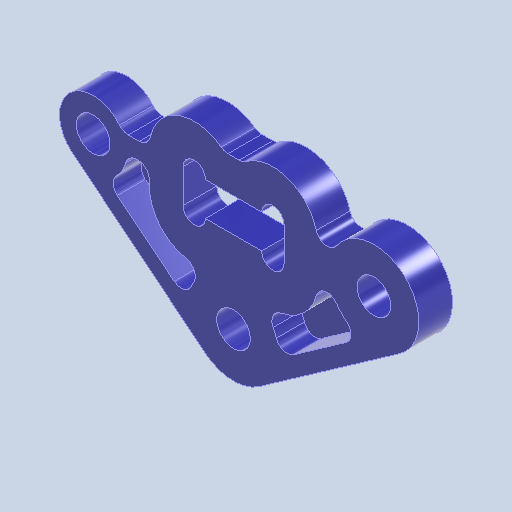
# Autodesk Inventor part: 足 横wing固定用外フレーム
Saved by Autodesk Inventor 2023.1 (Build 271208000, 208)
## iProperties
Created: 2020-05-17
Part Number: 足 横wing固定用外フレーム
Material: アルミニウム 2014-T6
Document SubType Name: Modeling
Designer: mozar
Density: 2.78927 g/cm^3
Appearance: 滑らか - 濃紺色
Mass: 2.27772 g
Surface Area: 11.4754 cm^2
Volume: 0.8166 cm^3
Author: mozar
Autodesk Inventor part; units mm, degrees
ref_plane "YZ Plane" through (0, 0, 0) normal (1, 0, 0) x (0, 1, 0)
ref_plane "XZ Plane" through (0, 0, 0) normal (0, 1, 0) x (-1, 0, 0)
ref_plane "XY Plane" through (0, 0, 0) normal (0, 0, 1) x (1, 0, 0)
sketch "スケッチ1" plane through (0, 0, 0) normal (0, 0, 1) x (1, 0, 0)
  arc A0 (-67.3471, 114.501) -> (-65.1952, 116.9091) centre (-69, 118.1435) ccw
  line L0 (-67.3471, 114.501) -> (-45.8039, 94.0088)
  line L1 (-45.8039, 94.0088) -> (-41.2946, 99.2468)
  arc A1 (-42.0113, 103.4843) -> (-41.2946, 99.2468) centre (-38.3264, 101.9283) ccw
  line L2 (-42.0113, 103.4843) -> (-65.1952, 116.9091)
  circle A2 centre (-69, 118.1435) radius 1.5
  line L3 (-8.5314, 132.4283) -> (8.5314, 132.4283)
  arc A3 (8.9906, 133.8477) -> (8.5314, 132.4283) centre (12.5, 131.9283) ccw
  line L4 (8.9906, 133.8477) -> (-8.0073, 147.851)
  arc A4 (-12.2806, 145.8755) -> (-8.0073, 147.851) centre (-12.9215, 152.8712) ccw
  line L5 (-12.2806, 145.8755) -> (-12.08, 135.9062)
  arc A5 (-8.5314, 132.4283) -> (-12.08, 135.9062) centre (-12.5, 131.9283) ccw
  line L6 (-40.5367, 98.5944) -> (-45.0784, 93.3188)
  line L7 (-45.0784, 93.3188) -> (-23.1821, 72.4907)
  arc A6 (-21.219, 73.2225) -> (-23.1821, 72.4907) centre (-20.8522, 69.2393) ccw
  line L8 (-21.219, 73.2225) -> (-20.9998, 79.7658)
  arc A7 (-26.8226, 92.2649) -> (-20.9998, 79.7658) centre (-20.2328, 87.729) ccw
  line L9 (-26.8226, 92.2649) -> (-35.513, 99.0849)
  arc A8 (-40.5367, 98.5944) -> (-35.513, 99.0849) centre (-38.3264, 101.9283) ccw
  line L10 (-53.762, 124.0122) -> (-40.2555, 105.4324)
  arc A9 (-36.7463, 105.603) -> (-40.2555, 105.4324) centre (-38.3264, 101.9283) ccw
  arc A10 (-36.7463, 105.603) -> (-35.5935, 105.8692) centre (-36.3513, 106.5217) ccw
  line L11 (-35.5935, 105.8692) -> (-15.9908, 128.6398)
  arc A11 (-15.9908, 128.6398) -> (-15.8989, 129.8194) centre (-16.7486, 129.2922) ccw
  arc A12 (-16.3868, 130.9834) -> (-15.8989, 129.8194) centre (-12.5, 131.9283) ccw
  line L12 (-16.3868, 130.9834) -> (-52.5003, 126.8796)
  arc A13 (-53.762, 124.0122) -> (-52.5003, 126.8796) centre (-56.5, 126.9283) ccw
  line L13 (-20.101, 159.5757) -> (-51.6361, 130.4057)
  line L14 (-51.6361, 130.4057) -> (-19.1983, 149.7164)
  arc A14 (-18.3334, 157.3502) -> (-19.1983, 149.7164) centre (-12.9215, 152.8712) ccw
  arc A15 (-18.3334, 157.3502) -> (-18.8282, 158.9491) centre (-19.1038, 157.9878) ccw
  arc A16 (-20.101, 159.5757) -> (-18.8282, 158.9491) centre (-17.726, 162.7942) ccw
  line L15 (-52.6132, 127.8732) -> (-16.4997, 131.977)
  arc A17 (-13.0798, 135.886) -> (-16.4997, 131.977) centre (-12.5, 131.9283) ccw
  line L16 (-13.0798, 135.886) -> (-13.2804, 145.8553)
  arc A18 (-18.6867, 148.8571) -> (-13.2804, 145.8553) centre (-12.9215, 152.8712) ccw
  line L17 (-18.6867, 148.8571) -> (-52.8341, 128.5287)
  arc A19 (-52.6132, 127.8732) -> (-52.8341, 128.5287) centre (-56.5, 126.9283) ccw
  line L18 (-41.0644, 104.8444) -> (-54.5709, 123.4242)
  arc A20 (-57.3125, 123.0117) -> (-54.5709, 123.4242) centre (-56.5, 126.9283) ccw
  arc A21 (-63.1458, 122.4283) -> (-57.3125, 123.0117) centre (-60.5, 125.4283) ccw
  line L19 (-63.1458, 122.4283) -> (-66.7175, 122.4283)
  arc A22 (-66.7175, 122.4283) -> (-67.6036, 121.8918) centre (-66.7175, 121.4283) ccw
  arc A23 (-65.0045, 117.9542) -> (-67.6036, 121.8918) centre (-69, 118.1435) ccw
  line L20 (-65.0045, 117.9542) -> (-41.5102, 104.3497)
  arc A24 (-41.0644, 104.8444) -> (-41.5102, 104.3497) centre (-38.3264, 101.9283) ccw
  circle A25 centre (20.2328, 87.729) radius 5.75
  circle A26 centre (-20.2328, 87.729) radius 5.75
  circle A27 centre (-20.8522, 69.2393) radius 1.5
  circle A28 centre (-19.5, 53.0338) radius 1.5
  line L21 (-19.7781, 65.3862) -> (-19.5876, 63.104)
  line L22 (-19.5876, 63.104) -> (-7.2173, 67.5101)
  arc A29 (-5.9007, 74.1795) -> (-7.2173, 67.5101) centre (0, 69.55) ccw
  line L23 (-5.9007, 74.1795) -> (-14.6278, 82.0207)
  arc A30 (-20.0004, 79.7323) -> (-14.6278, 82.0207) centre (-20.2328, 87.729) ccw
  line L24 (-20.0004, 79.7323) -> (-20.2196, 73.189)
  arc A31 (-19.7781, 65.3862) -> (-20.2196, 73.189) centre (-20.8522, 69.2393) ccw
  circle A32 centre (-17.726, 162.7942) radius 1.5
  circle A33 centre (-12.9215, 152.8712) radius 4.025
  line L25 (-34.7337, 103.6868) -> (-0.8086, 115.3011)
  line L26 (-0.8086, 115.3011) -> (-10.5399, 128.4414)
  arc A34 (-14.0801, 128.2536) -> (-10.5399, 128.4414) centre (-12.5, 131.9283) ccw
  arc A35 (-14.0801, 128.2536) -> (-15.2329, 127.9873) centre (-14.4751, 127.3349) ccw
  line L27 (-15.2329, 127.9873) -> (-34.8356, 105.2168)
  arc A36 (-34.8356, 105.2168) -> (-34.9275, 104.0372) centre (-34.0778, 104.5644) ccw
  arc A37 (-34.7337, 103.6868) -> (-34.9275, 104.0372) centre (-38.3264, 101.9283) ccw
  line L28 (0.8086, 115.3011) -> (34.7337, 103.6868)
  arc A38 (35.1946, 104.4166) -> (34.7337, 103.6868) centre (38.3264, 101.9283) ccw
  line L29 (35.1946, 104.4166) -> (14.9874, 127.8894)
  arc A39 (14.9874, 127.8894) -> (13.8836, 128.1752) centre (14.2295, 127.2369) ccw
  arc A40 (10.5399, 128.4414) -> (13.8836, 128.1752) centre (12.5, 131.9283) ccw
  line L30 (10.5399, 128.4414) -> (0.8086, 115.3011)
  line L31 (34.4098, 102.7407) -> (1.3578, 114.0561)
  line L32 (1.3578, 114.0561) -> (15.8828, 94.4429)
  arc A41 (26.2052, 93.0515) -> (15.8828, 94.4429) centre (20.2328, 87.729) ccw
  line L33 (26.2052, 93.0515) -> (34.8957, 99.8715)
  arc A42 (34.4098, 102.7407) -> (34.8957, 99.8715) centre (38.3264, 101.9283) ccw
  line L34 (0, 114.2093) -> (-15.0792, 93.8478)
  arc A43 (-12.2484, 88.229) -> (-15.0792, 93.8478) centre (-20.2328, 87.729) ccw
  line L35 (-12.2484, 88.229) -> (12.2484, 88.229)
  arc A44 (15.0792, 93.8478) -> (12.2484, 88.229) centre (20.2328, 87.729) ccw
  line L36 (15.0792, 93.8478) -> (0, 114.2093)
  line L37 (0, 115.8896) -> (9.7363, 129.0366)
  arc A45 (8.753, 130.5283) -> (9.7363, 129.0366) centre (12.5, 131.9283) ccw
  arc A46 (8.753, 130.5283) -> (7.8163, 131.1783) centre (7.8163, 130.1783) ccw
  line L38 (7.8163, 131.1783) -> (-7.8163, 131.1783)
  arc A47 (-7.8163, 131.1783) -> (-8.753, 130.5283) centre (-7.8163, 130.1783) ccw
  arc A48 (-9.7363, 129.0366) -> (-8.753, 130.5283) centre (-12.5, 131.9283) ccw
  line L39 (-9.7363, 129.0366) -> (0, 115.8896)
  circle A49 centre (-12.5, 131.9283) radius 1.5
  line L40 (-34.8957, 99.8715) -> (-26.2052, 93.0515)
  arc A50 (-15.8828, 94.4429) -> (-26.2052, 93.0515) centre (-20.2328, 87.729) ccw
  line L41 (-15.8828, 94.4429) -> (-1.3578, 114.0561)
  line L42 (-1.3578, 114.0561) -> (-34.4098, 102.7407)
  arc A51 (-34.8957, 99.8715) -> (-34.4098, 102.7407) centre (-38.3264, 101.9283) ccw
  line L43 (42.9737, 57.5032) -> (38.0562, 97.9374)
  arc A52 (35.513, 99.0849) -> (38.0562, 97.9374) centre (38.3264, 101.9283) ccw
  line L44 (35.513, 99.0849) -> (26.8226, 92.2649)
  arc A53 (25.202, 81.4595) -> (26.8226, 92.2649) centre (20.2328, 87.729) ccw
  line L45 (25.202, 81.4595) -> (42.111, 57.1462)
  arc A54 (42.9737, 57.5032) -> (42.111, 57.1462) centre (44.2539, 53.1892) ccw
  arc A55 (-13.9594, 82.7646) -> (-12.2484, 87.229) centre (-20.2328, 87.729) ccw
  line L46 (-13.9594, 82.7646) -> (-5.2323, 74.9234)
  arc A56 (5.2323, 74.9234) -> (-5.2323, 74.9234) centre (0, 69.55) ccw
  line L47 (5.2323, 74.9234) -> (13.9594, 82.7646)
  arc A57 (12.2484, 87.229) -> (13.9594, 82.7646) centre (20.2328, 87.729) ccw
  line L48 (12.2484, 87.229) -> (-12.2484, 87.229)
  line L49 (7.1924, 67.424) -> (40.2326, 55.2089)
  arc A58 (41.29, 56.5752) -> (40.2326, 55.2089) centre (44.2539, 53.1892) ccw
  line L50 (41.29, 56.5752) -> (24.381, 80.8885)
  arc A59 (14.6278, 82.0207) -> (24.381, 80.8885) centre (20.2328, 87.729) ccw
  line L51 (14.6278, 82.0207) -> (5.9007, 74.1795)
  arc A60 (7.1924, 67.424) -> (5.9007, 74.1795) centre (0, 69.55) ccw
  circle A61 centre (0, 69.55) radius 4.5
  arc A62 (-1.9, 54.6661) -> (-0.5, 55.5826) centre (-1.5, 55.5826) ccw
  line L52 (-0.5, 55.5826) -> (-0.5, 61.1834)
  arc A63 (-0.5, 61.1834) -> (-1.3235, 62.1677) centre (-1.5, 61.1834) ccw
  arc A64 (-6.8817, 66.5681) -> (-1.3235, 62.1677) centre (0, 69.55) ccw
  line L53 (-6.8817, 66.5681) -> (-19.5016, 62.0731)
  line L54 (-19.5016, 62.0731) -> (-19.0793, 57.0116)
  arc A65 (-15.8112, 51.487) -> (-19.0793, 57.0116) centre (-19.5, 53.0338) ccw
  arc A66 (-15.8112, 51.487) -> (-11.0422, 51.0882) centre (-7.5, 122.1642) ccw
  arc A67 (-8.1719, 51.9865) -> (-11.0422, 51.0882) centre (-8.5, 48) ccw
  arc A68 (-8.1719, 51.9865) -> (-7.1719, 52.5865) centre (-8.0899, 52.9832) ccw
  arc A69 (-1.9, 54.6661) -> (-7.1719, 52.5865) centre (-3.5, 51) ccw
  circle A70 centre (44.2539, 53.1892) radius 1.5
  arc A71 (10.9, 51.2) -> (11.5, 51) centre (11.5, 52) ccw
  line L55 (11.5, 51) -> (11.6438, 51)
  arc A72 (11.6438, 51) -> (12.2438, 51.2) centre (11.6438, 52) ccw
  arc A73 (14.9719, 51.9865) -> (12.2438, 51.2) centre (14.6438, 48) ccw
  arc A74 (14.9719, 51.9865) -> (15.9719, 52.5865) centre (15.0539, 52.9832) ccw
  arc A75 (22.2896, 54) -> (15.9719, 52.5865) centre (19.6438, 51) ccw
  line L56 (22.2896, 54) -> (23.9981, 54)
  arc A76 (30.5528, 51.8483) -> (23.9981, 54) centre (26.6438, 51) ccw
  arc A77 (33.5683, 51.5066) -> (30.5528, 51.8483) centre (31.6438, 48) ccw
  arc A78 (33.5683, 51.5066) -> (34.4381, 51) centre (34.4381, 52) ccw
  line L57 (34.4381, 51) -> (35.1308, 51)
  arc A79 (35.1308, 51) -> (35.5246, 51.0808) centre (35.1308, 52) ccw
  line L58 (35.5246, 51.0808) -> (39.1601, 52.6385)
  arc A80 (39.1601, 52.6385) -> (39.764, 53.4907) centre (38.7663, 53.5577) ccw
  arc A81 (39.8859, 54.271) -> (39.764, 53.4907) centre (44.2539, 53.1892) ccw
  line L59 (39.8859, 54.271) -> (6.8456, 66.4861)
  arc A82 (1.3235, 62.1677) -> (6.8456, 66.4861) centre (0, 69.55) ccw
  arc A83 (1.3235, 62.1677) -> (0.5, 61.1834) centre (1.5, 61.1834) ccw
  line L60 (0.5, 61.1834) -> (0.5, 55.5826)
  arc A84 (0.5, 55.5826) -> (1.9, 54.6661) centre (1.5, 55.5826) ccw
  arc A85 (7.1719, 52.5865) -> (1.9, 54.6661) centre (3.5, 51) ccw
  arc A86 (7.1719, 52.5865) -> (8.1719, 51.9865) centre (8.0899, 52.9832) ccw
  arc A87 (10.9, 51.2) -> (8.1719, 51.9865) centre (8.5, 48) ccw
  arc A88 (9.5, 48) -> (7.5, 48) centre (8.5, 48) ccw
  line L61 (7.5, 48) -> (7.5, 45)
  line L62 (7.5, 45) -> (-7.5, 45)
  line L63 (-7.5, 45) -> (-7.5, 48)
  arc A89 (-7.5, 48) -> (-9.4996, 48.027) centre (-8.5, 48) ccw
  arc A90 (-20.1841, 49.0927) -> (-9.4996, 48.027) centre (-7.5, 122.1642) ccw
  arc A91 (-20.5741, 56.8869) -> (-20.1841, 49.0927) centre (-19.5, 53.0338) ccw
  line L64 (-20.5741, 56.8869) -> (-21.2729, 65.2615)
  arc A92 (-24.2159, 71.4039) -> (-21.2729, 65.2615) centre (-20.8522, 69.2393) ccw
  line L65 (-24.2159, 71.4039) -> (-69.1506, 114.1463)
  arc A93 (-72.9846, 117.7933) -> (-69.1506, 114.1463) centre (-69, 118.1435) ccw
  line L66 (-72.9846, 117.7933) -> (-76.8602, 121.4798)
  arc A94 (-81.2136, 123.942) -> (-76.8602, 121.4798) centre (-77.5, 125.4283) ccw
  arc A95 (-81.2136, 129.9146) -> (-81.2136, 123.942) centre (-81.5, 126.9283) ccw
  arc A96 (-74.8542, 131.4283) -> (-81.2136, 129.9146) centre (-77.5, 128.4283) ccw
  line L67 (-74.8542, 131.4283) -> (-63.1458, 131.4283)
  arc A97 (-57.3125, 130.8449) -> (-63.1458, 131.4283) centre (-60.5, 128.4283) ccw
  arc A98 (-54.125, 130.1469) -> (-57.3125, 130.8449) centre (-56.5, 126.9283) ccw
  line L68 (-54.125, 130.1469) -> (-21.1196, 160.6768)
  arc A99 (-14.0261, 161.2742) -> (-21.1196, 160.6768) centre (-17.726, 162.7942) ccw
  arc A100 (-14.0261, 161.2742) -> (-13.0787, 159.8944) centre (-13.1011, 160.8942) ccw
  arc A101 (-7.0536, 149.0088) -> (-13.0787, 159.8944) centre (-12.9215, 152.8712) ccw
  line L69 (-7.0536, 149.0088) -> (9.9444, 135.0054)
  arc A102 (16.0056, 130.002) -> (9.9444, 135.0054) centre (12.5, 131.9283) ccw
  arc A103 (16.0056, 130.002) -> (16.1242, 128.868) centre (16.882, 129.5204) ccw
  line L70 (16.1242, 128.868) -> (35.839, 105.9672)
  arc A104 (35.839, 105.9672) -> (36.9428, 105.6814) centre (36.5969, 106.6196) ccw
  arc A105 (39.5453, 98.1185) -> (36.9428, 105.6814) centre (38.3264, 101.9283) ccw
  line L71 (39.5453, 98.1185) -> (44.4627, 57.6843)
  arc A106 (41.3752, 49.7304) -> (44.4627, 57.6843) centre (44.2539, 53.1892) ccw
  arc A107 (41.3752, 49.7304) -> (40.3416, 49.881) centre (40.7355, 48.9618) ccw
  line L72 (40.3416, 49.881) -> (36.2346, 48.1212)
  arc A108 (35.6438, 48) -> (36.2346, 48.1212) centre (35.6438, 49.5) ccw
  line L73 (35.6438, 48) -> (32.6438, 48)
  arc A109 (32.6438, 48) -> (30.6438, 48) centre (31.6438, 48) ccw
  line L74 (30.6438, 48) -> (30.6438, 45)
  line L75 (30.6438, 45) -> (15.6438, 45)
  line L76 (15.6438, 45) -> (15.6438, 48)
  arc A110 (15.6438, 48) -> (13.6438, 48) centre (14.6438, 48) ccw
  line L77 (13.6438, 48) -> (9.5, 48)
  line L78 (18.6438, 51) -> (18.6438, 48)
  arc A111 (18.6438, 48) -> (20.6438, 48) centre (19.6438, 48) ccw
  line L79 (20.6438, 48) -> (25.6438, 48)
  arc A112 (25.6438, 48) -> (27.6438, 48) centre (26.6438, 48) ccw
  line L80 (27.6438, 48) -> (27.6438, 51)
  arc A113 (27.6438, 51) -> (25.6438, 51) centre (26.6438, 51) ccw
  line L81 (25.6438, 51) -> (20.6438, 51)
  arc A114 (20.6438, 51) -> (18.6438, 51) centre (19.6438, 51) ccw
  line L82 (-4.5, 51) -> (-4.5, 48)
  arc A115 (-4.5, 48) -> (-2.5, 48) centre (-3.5, 48) ccw
  line L83 (-2.5, 48) -> (2.5, 48)
  arc A116 (2.5, 48) -> (4.5, 48) centre (3.5, 48) ccw
  line L84 (4.5, 48) -> (4.5, 51)
  arc A117 (4.5, 51) -> (2.5, 51) centre (3.5, 51) ccw
  line L85 (2.5, 51) -> (-2.5, 51)
  arc A118 (-2.5, 51) -> (-4.5, 51) centre (-3.5, 51) ccw
  circle A119 centre (12.5, 131.9283) radius 1.5
  circle A120 centre (-38.3264, 101.9283) radius 1.5
  circle A121 centre (38.3264, 101.9283) radius 1.5
  arc A122 (42.1775, 57.1816) -> (42.1571, 57.1709) centre (44.2546, 53.1897) ccw
  line L86 (42.1571, 57.1709) -> (42.1563, 57.1713)
  arc A123 (42.1563, 57.1713) -> (42.1775, 57.1816) centre (41.7307, 58.0762) ccw
  circle A124 centre (-56.5, 126.9283) radius 1.5
  circle A125 centre (-81.5, 126.9283) radius 1.5
  line L87 (-78.5, 128.4283) -> (-78.5, 125.4283)
  arc A126 (-78.5, 125.4283) -> (-76.5, 125.4283) centre (-77.5, 125.4283) ccw
  line L88 (-76.5, 125.4283) -> (-61.5, 125.4283)
  arc A127 (-61.5, 125.4283) -> (-59.5, 125.4283) centre (-60.5, 125.4283) ccw
  line L89 (-59.5, 125.4283) -> (-59.5, 128.4283)
  arc A128 (-59.5, 128.4283) -> (-61.5, 128.4283) centre (-60.5, 128.4283) ccw
  line L90 (-61.5, 128.4283) -> (-76.5, 128.4283)
  arc A129 (-76.5, 128.4283) -> (-78.5, 128.4283) centre (-77.5, 128.4283) ccw
  line L91 (-69, 118.1435) -> (-56.5, 126.9283) construction
  line L92 (-68.5688, 117.5298) -> (-56.0688, 126.3147)
  line L93 (-56.9312, 127.5419) -> (-69.4312, 118.7571)
  arc A130 (-69.4312, 118.7571) -> (-68.5688, 117.5298) centre (-69, 118.1435) ccw
  arc A131 (-56.0688, 126.3147) -> (-56.9312, 127.5419) centre (-56.5, 126.9283) ccw
  line L94 (-81.5, 126.9283) -> (-69, 118.1435) construction
  line L95 (-81.9312, 126.3147) -> (-69.4312, 117.5298)
  line L96 (-68.5688, 118.7571) -> (-81.0688, 127.5419)
  arc A132 (-81.0688, 127.5419) -> (-81.9312, 126.3147) centre (-81.5, 126.9283) ccw
  arc A133 (-69.4312, 117.5298) -> (-68.5688, 118.7571) centre (-69, 118.1435) ccw
  line L97 (-63.1458, 122.4283) -> (-74.8542, 122.4283)
  arc A134 (-81.5, 125.4283) -> (-74.8542, 122.4283) centre (-77.5, 125.4283) ccw
  line L98 (-81.5, 125.4283) -> (-81.5, 128.4283)
  arc A135 (-74.8542, 131.4283) -> (-81.5, 128.4283) centre (-77.5, 128.4283) ccw
  line L99 (-74.8542, 131.4283) -> (-63.1458, 131.4283)
  arc A136 (-56.5, 128.4283) -> (-63.1458, 131.4283) centre (-60.5, 128.4283) ccw
  line L100 (-56.5, 128.4283) -> (-56.5, 125.4283)
  arc A137 (-63.1458, 122.4283) -> (-56.5, 125.4283) centre (-60.5, 125.4283) ccw
  circle A138 centre (-56.5, 126.9283) radius 4
  circle A139 centre (-69, 118.1435) radius 4
  point P0 (0, 0)
  point P1 (0, 0)
  point P2 (-62.75, 122.5359)
  point P3 (-75.25, 122.5359)
  point P4 (-62.3651, 121.8897)
  point P5 (-75.6349, 121.8897)
  point P6 (-72.6458, 119.789)
  point P7 (-67.3471, 114.501)
  point P8 (-65.1952, 116.9091)
  point P9 (-65.3542, 119.789)
  dimension "d0" = 1.5
  dimension "d1" = 1.5
  dimension "d2" = 3
  constraints: 246 point on circle, 206 end point, 138 centre point, 19 horizontal, 12 vertical, 8 tangent, 2 coincident, 2 midpoint, 2 parallel, 1 concentric, 541 other
  measures "d0" diameter of A131
  measures "d1" diameter of A133
  measures "d2" distance between parallel lines of L88 L97
extrude "押し出し2" add sketch "スケッチ1" against normal blind 3 contours A139 A93 L95 A2 L92 A23 A0 | A94 A134 A125 L95 | A139 L96 A2 L95 | L95 A134 L97 L96 A139 | L92 A2 L93 A23 | A23 L93 L19 A21 L92 | A95 A135 A125 A134 | L95 A125 L96 L87 A126 L97 A134 | L95 A130 L92 A2 | A2 L96 L93 A130 L95 | A139 A23 L93 A2 L96 | L96 L97 A22 A139 | A23 A22 L19 L93 | L92 A133 L96 L93 A2 | L92 A138 A21 | A21 L19 L93 A127 A138 L92 | A20 A137 A124 A136 A98 A138 A19 A13 | A96 L67 A97 A138 A128 L90 A129 L87 L96 A125 A135 | L98 L95 A125 | A125 L98 A132 L95 | L95 L98 A132 L96 A125 | A2 L93 L96 | A130 L93 L96 A133 | L96 A126 L88 A127 L93 L19 L97 | A138 L92 A124 A137 | A138 A127 L89 L93 A124 L92 | A125 L96 A132 L98 | L95 A132 L98 | L100 L92 A131 A124 | A124 L92 L100 | A124 L93 A131 L100 L92 | L100 A131 L92 | L93 L89 A128 A138 A136 A124 | A124 L100 A131 L93
sketch "スケッチ2" plane through (0, 0, 0) normal (0, 0, 1) x (1, 0, 0)
  line L0 (-76.5, 125.4283) -> (-61.5, 125.4283) projected
  arc A0 (-61.5, 125.4283) -> (-59.5, 125.4283) centre (-60.5, 125.4283) ccw projected
  line L1 (-59.5, 125.4283) -> (-59.5, 128.4283) projected
  arc A1 (-59.5, 128.4283) -> (-61.5, 128.4283) centre (-60.5, 128.4283) ccw projected
  line L2 (-61.5, 128.4283) -> (-76.5, 128.4283) projected
  arc A2 (-76.5, 128.4283) -> (-78.5, 128.4283) centre (-77.5, 128.4283) ccw projected
  line L3 (-78.5, 128.4283) -> (-78.5, 125.4283) projected
  arc A3 (-78.5, 125.4283) -> (-76.5, 125.4283) centre (-77.5, 125.4283) ccw projected
  line L4 (-72.6458, 119.789) -> (-75.6349, 121.8897) projected
  arc A4 (-81.2136, 123.942) -> (-75.6349, 121.8897) centre (-77.5, 125.4283) ccw projected
  arc A5 (-81.2136, 129.9146) -> (-81.2136, 123.942) centre (-81.5, 126.9283) ccw projected
  arc A6 (-74.8542, 131.4283) -> (-81.2136, 129.9146) centre (-77.5, 128.4283) ccw projected
  line L5 (-74.8542, 131.4283) -> (-63.1458, 131.4283) projected
  arc A7 (-57.3125, 130.8449) -> (-63.1458, 131.4283) centre (-60.5, 128.4283) ccw projected
  arc A8 (-57.3125, 123.0117) -> (-57.3125, 130.8449) centre (-56.5, 126.9283) ccw projected
  arc A9 (-62.3651, 121.8897) -> (-57.3125, 123.0117) centre (-60.5, 125.4283) ccw projected
  line L6 (-62.3651, 121.8897) -> (-65.3542, 119.789) projected
  arc A10 (-72.6458, 119.789) -> (-65.3542, 119.789) centre (-69, 118.1435) ccw projected
  point P0 (0, 0)
hole "穴1" at (-56.5, 126.9283, 0) at (-81.5, 126.9283, 0) at (-69, 118.1435, 0) direction (0, 0, -1) diameter 3 depth 12 tip angle 118
fillet "フィレット1" radius 1 10 edges at (-62.3651, 121.8897, -1.5) (-57.3125, 123.0117, -1.5) (-65.3542, 119.789, -1.5) (-57.3125, 130.8449, -1.5) (-72.6458, 119.789, -1.5) (-75.6349, 121.8897, -1.5) (-63.1458, 131.4283, -1.5) (-81.2136, 123.942, -1.5) (-74.8542, 131.4283, -1.5) (-81.2136, 129.9146, -1.5)
sketch "スケッチ3" plane through (0, 0, 0) normal (0, 0, 1) x (1, 0, 0)
  arc A0 (-80.9707, 123.4398) -> (-81.7538, 123.939) centre (-81.8384, 122.9426) ccw projected
  arc A1 (-81.7538, 129.9175) -> (-81.7538, 123.939) centre (-81.5, 126.9283) ccw projected
  arc A2 (-81.7538, 129.9175) -> (-80.9707, 130.4168) centre (-81.8384, 130.9139) ccw projected
  arc A3 (-75.1, 131.6283) -> (-80.9707, 130.4168) centre (-77.5, 128.4283) ccw projected
  arc A4 (-75.1, 131.6283) -> (-74.5, 131.4283) centre (-74.5, 132.4283) ccw projected
  line L0 (-74.5, 131.4283) -> (-63.5, 131.4283) projected
  arc A5 (-63.5, 131.4283) -> (-62.9, 131.6283) centre (-63.5, 132.4283) ccw projected
  arc A6 (-57.6301, 131.2146) -> (-62.9, 131.6283) centre (-60.5, 128.4283) ccw projected
  arc A7 (-57.6301, 131.2146) -> (-56.8301, 130.9146) centre (-56.9126, 131.9112) ccw projected
  arc A8 (-56.8301, 122.9419) -> (-56.8301, 130.9146) centre (-56.5, 126.9283) ccw projected
  arc A9 (-56.8301, 122.9419) -> (-57.6301, 122.6419) centre (-56.9126, 121.9453) ccw projected
  arc A10 (-61.9028, 121.6823) -> (-57.6301, 122.6419) centre (-60.5, 125.4283) ccw projected
  arc A11 (-61.9028, 121.6823) -> (-62.8285, 121.564) centre (-62.2535, 120.7458) ccw projected
  line L1 (-62.8285, 121.564) -> (-64.7367, 120.223) projected
  arc A12 (-64.7367, 120.223) -> (-65.1294, 119.1525) centre (-64.1617, 119.4048) ccw projected
  arc A13 (-72.8706, 119.1525) -> (-65.1294, 119.1525) centre (-69, 118.1435) ccw projected
  arc A14 (-72.8706, 119.1525) -> (-73.2633, 120.223) centre (-73.8383, 119.4048) ccw projected
  line L2 (-73.2633, 120.223) -> (-75.1715, 121.564) projected
  arc A15 (-75.1715, 121.564) -> (-76.0972, 121.6823) centre (-75.7465, 120.7458) ccw projected
  arc A16 (-80.9707, 123.4398) -> (-76.0972, 121.6823) centre (-77.5, 125.4283) ccw projected
  circle A17 centre (-81.5, 126.9283) radius 1.5 projected
  circle A18 centre (-56.5, 126.9283) radius 1.5 projected
  circle A19 centre (-69, 118.1435) radius 1.5 projected
  line L3 (-76.5, 125.4283) -> (-61.5, 125.4283) projected
  arc A20 (-61.5, 125.4283) -> (-59.5, 125.4283) centre (-60.5, 125.4283) ccw projected
  line L4 (-59.5, 125.4283) -> (-59.5, 128.4283) projected
  arc A21 (-59.5, 128.4283) -> (-61.5, 128.4283) centre (-60.5, 128.4283) ccw projected
  line L5 (-61.5, 128.4283) -> (-76.5, 128.4283) projected
  arc A22 (-76.5, 128.4283) -> (-78.5, 128.4283) centre (-77.5, 128.4283) ccw projected
  line L6 (-78.5, 128.4283) -> (-78.5, 125.4283) projected
  arc A23 (-78.5, 125.4283) -> (-76.5, 125.4283) centre (-77.5, 125.4283) ccw projected
  line L7 (-76.5, 128.4283) -> (-61.5, 128.4283) projected
  line L8 (-73.5, 128.4283) -> (-64.5, 128.4283)
  line L9 (-64.5, 128.4283) -> (-64.5, 125.4283)
  line L10 (-64.5, 125.4283) -> (-73.5, 125.4283)
  line L11 (-73.5, 125.4283) -> (-73.5, 128.4283)
  circle A24 centre (-72.5, 128.4283) radius 1
  circle A25 centre (-65.5, 128.4283) radius 1
  circle A26 centre (-65.5, 125.4283) radius 1
  line L12 (-61.5, 125.4283) -> (-76.5, 125.4283) projected
  circle A27 centre (-72.5, 125.4283) radius 1
  line L13 (-61.5, 131.4283) -> (-76.5, 131.4283)
  line L14 (-76.5, 131.4283) -> (-76.5, 122.4283)
  line L15 (-76.5, 122.4283) -> (-61.5, 122.4283)
  line L16 (-61.5, 122.4283) -> (-61.5, 131.4283)
  circle A28 centre (-72.5, 128.4283) radius 4
  circle A29 centre (-65.5, 128.4283) radius 4
  circle A30 centre (-72.5, 125.4283) radius 4
  circle A31 centre (-65.5, 125.4283) radius 4
  arc A32 (-81.7538, 129.9175) -> (-81.7538, 123.939) centre (-81.5, 126.9283) ccw projected
  circle A33 centre (-81.5, 126.9283) radius 3
  circle A34 centre (-69, 118.1435) radius 4
  line L17 (-81.5, 126.9283) -> (-69, 118.1435) construction
  line L18 (-81.9312, 126.3147) -> (-69.4312, 117.5298)
  line L19 (-68.5688, 118.7571) -> (-81.0688, 127.5419)
  arc A35 (-81.0688, 127.5419) -> (-81.9312, 126.3147) centre (-81.5, 126.9283) ccw
  arc A36 (-69.4312, 117.5298) -> (-68.5688, 118.7571) centre (-69, 118.1435) ccw
  line L20 (-69, 118.1435) -> (-56.5, 126.9283) construction
  line L21 (-68.5688, 117.5298) -> (-56.0688, 126.3147)
  line L22 (-56.9312, 127.5419) -> (-69.4312, 118.7571)
  arc A37 (-69.4312, 118.7571) -> (-68.5688, 117.5298) centre (-69, 118.1435) ccw
  arc A38 (-56.0688, 126.3147) -> (-56.9312, 127.5419) centre (-56.5, 126.9283) ccw
  circle A39 centre (-81.5, 126.9283) radius 1.5 projected
  line L23 (-56.5, 126.9283) -> (-81.5, 126.9283) construction
  line L24 (-56.5, 128.4283) -> (-81.5, 128.4283)
  line L25 (-81.5, 125.4283) -> (-56.5, 125.4283)
  arc A40 (-56.5, 125.4283) -> (-56.5, 128.4283) centre (-56.5, 126.9283) ccw
  arc A41 (-81.5, 128.4283) -> (-81.5, 125.4283) centre (-81.5, 126.9283) ccw
  arc A42 (-56.8301, 122.9419) -> (-56.8301, 130.9146) centre (-56.5, 126.9283) ccw projected
  circle A43 centre (-56.5, 126.9283) radius 4
  point P0 (0, 0)
  point P1 (-69, 128.4283)
  point P2 (-75.25, 122.5359)
  point P3 (-62.75, 122.5359)
  point P4 (-69, 126.9283)
  point P5 (-63.0084, 131.5575)
  point P6 (-59.8191, 129.1607)
  point P7 (-78.9019, 128.4283)
  point P8 (-74.9916, 131.5575)
  point P9 (-79.5547, 124.6445)
  point P10 (-59.2834, 124.0555)
  point P11 (-61.5, 122.4977)
  point P12 (-61.5987, 122.4283)
  point P13 (-62.8285, 121.564)
  point P14 (-68.1458, 131.4283)
  point P15 (-69.8542, 131.4283)
  point P16 (-60.2081, 128.4283)
  dimension "d15" = 9
  dimension "d16" = 3
  dimension "d17" = 2
  dimension "d18" = 2
  dimension "d19" = 2
  dimension "d20" = 2
  dimension "d21" = 3
  dimension "d22" = 3
  dimension "d23" = 3
  dimension "d24" = 3
  dimension "d25" = 3
  dimension "d26" = 1.5
  dimension "d27" = 1.5
  dimension "d28" = 3
  constraints: 40 end point, 16 tangent, 14 centre point, 12 point on circle, 7 parallel, 5 midpoint, 5 point on line, 3 coincident, 2 horizontal, 2 perpendicular, 12 other
  measures "d15" distance of L9.end L10.end
  measures "d16" distance of L8.end L9.end
  measures "d17" diameter of A24
  measures "d18" diameter of A25
  measures "d19" diameter of A26
  measures "d20" diameter of A27
  measures "d21" distance between parallel lines of L8 L13
  measures "d22" radial gap between concentric circles of A24 A28
  measures "d23" radial gap between concentric circles of A25 A29
  measures "d24" radial gap between concentric circles of A27 A30
  measures "d25" radial gap between concentric circles of A26 A31
  measures "d26" diameter of A36
  measures "d27" diameter of A38
  measures "d28" diameter of A41
extrude "押し出し3" cut sketch "スケッチ3" against normal blind 10 contours A0 A33 L18 L14 L15 A15 A16 | A2 A3 A4 A28 L13 L14 A22 L24 A33 | L18 L15 L14 | L14 L13 A28 | A5 A6 A7 A43 A21 L16 L13 A29 | L21 L15 L16 A43 A9 A10 A11 | L13 L16 A29
extrude "押し出し4" add sketch "スケッチ3" against normal blind 3 contours L6 L24 L14 L25 L19 | L25 L19 A23 | L6 L19 L25 | A28 L0 A4 | L19 L25 A23 | A29 A5 L0 | L24 A43 L25 L16 | L25 A43 L22 A20 | L24 L4 L22 L25 A43 | L22 A43 A20 | L25 L22 A43 | A43 L22 L25 A20 | L22 L4 L25
extrude "押し出し5" add sketch "スケッチ3" against normal blind 3 contours A28 A30 L14 | L5 A30 A28 | A30 A28 L3 | L5 L11 L3 A28 A30 | A29 A31 L5 | L16 A31 A29 | L3 A29 A31 | A21 L24 A43 | A31 A29 L3 L9 L5 picked at (-59.9345, 128.5126)
extrude "押し出し6" cut sketch "スケッチ3" against normal blind 10 contours A24 L5 | L5 A24 | A27 L3 | L3 A27 | L21 L16 L15 | A25 L5 | L5 A25 | A26 L3 | L3 A26
fillet "フィレット2" radius 1 8 edges at (-79.5547, 124.6445, -1.5) (-78.9019, 128.4283, -1.5) (-59.2834, 124.0555, -1.5) (-76.5, 128.4283, -1.5) (-61.5, 128.4283, -1.5) (-60.2081, 128.4283, -1.5) (-69.8542, 131.4283, -1.5) (-68.1458, 131.4283, -1.5)
sketch "スケッチ4" plane through (0, 0, 0) normal (0, 0, 1) x (1, 0, 0)
  arc A0 (-68.5, 131.4283) -> (-67.9, 131.6283) centre (-68.5, 132.4283) ccw projected
  arc A1 (-61.6309, 129.4431) -> (-67.9, 131.6283) centre (-65.5, 128.4283) ccw projected
  arc A2 (-61.6309, 129.4431) -> (-59.8309, 129.1431) centre (-60.6636, 129.6968) ccw projected
  arc A3 (-58.7607, 123.6284) -> (-59.8309, 129.1431) centre (-56.5, 126.9283) ccw projected
  arc A4 (-58.7607, 123.6284) -> (-59.9008, 123.6215) centre (-59.3258, 122.8034) ccw projected
  line L0 (-59.9008, 123.6215) -> (-64.7367, 120.223) projected
  arc A5 (-64.7367, 120.223) -> (-65.1294, 119.1525) centre (-64.1617, 119.4048) ccw projected
  arc A6 (-72.8706, 119.1525) -> (-65.1294, 119.1525) centre (-69, 118.1435) ccw projected
  arc A7 (-72.8706, 119.1525) -> (-73.2633, 120.223) centre (-73.8383, 119.4048) ccw projected
  line L1 (-73.2633, 120.223) -> (-78.9884, 124.2465) projected
  arc A8 (-78.9884, 124.2465) -> (-80.0476, 124.3033) centre (-79.5634, 123.4283) ccw projected
  arc A9 (-79.1581, 128.8033) -> (-80.0476, 124.3033) centre (-81.5, 126.9283) ccw projected
  arc A10 (-79.1581, 128.8033) -> (-78.3775, 128.4283) centre (-78.3775, 129.4283) ccw projected
  line L2 (-78.3775, 128.4283) -> (-77.399, 128.4283) projected
  arc A11 (-77.399, 128.4283) -> (-76.4192, 129.2283) centre (-77.399, 129.4283) ccw projected
  arc A12 (-70.1, 131.6283) -> (-76.4192, 129.2283) centre (-72.5, 128.4283) ccw projected
  arc A13 (-70.1, 131.6283) -> (-69.5, 131.4283) centre (-69.5, 132.4283) ccw projected
  line L3 (-69.5, 131.4283) -> (-68.5, 131.4283) projected
  arc A14 (-64.5, 128.4283) -> (-66.5, 128.4283) centre (-65.5, 128.4283) ccw projected
  line L4 (-66.5, 128.4283) -> (-71.5, 128.4283) projected
  arc A15 (-71.5, 128.4283) -> (-73.5, 128.4283) centre (-72.5, 128.4283) ccw projected
  line L5 (-73.5, 128.4283) -> (-73.5, 125.4283) projected
  arc A16 (-73.5, 125.4283) -> (-71.5, 125.4283) centre (-72.5, 125.4283) ccw projected
  line L6 (-71.5, 125.4283) -> (-66.5, 125.4283) projected
  arc A17 (-66.5, 125.4283) -> (-64.5, 125.4283) centre (-65.5, 125.4283) ccw projected
  line L7 (-64.5, 125.4283) -> (-64.5, 128.4283) projected
  circle A18 centre (-81.5, 126.9283) radius 1.5 projected
  circle A19 centre (-56.5, 126.9283) radius 1.5 projected
  circle A20 centre (-69, 118.1435) radius 1.5 projected
  line L8 (-83.3819, 124.592) -> (-71.5092, 115.0284)
  arc A21 (-72.8706, 119.1525) -> (-65.1294, 119.1525) centre (-69, 118.1435) ccw projected
  line L9 (-66.7, 114.8708) -> (-54.2, 123.6556)
  arc A22 (-79.1581, 128.8033) -> (-80.0476, 124.3033) centre (-81.5, 126.9283) ccw projected
  point P0 (0, 0)
  constraints: 4 end point, 4 point on circle, 4 tangent
extrude "押し出し7" add sketch "スケッチ4" against normal blind 3 contours L9 A6 A5 L0 A4 A3 | L8 A9 A8 L1 A7 A6
sketch "スケッチ5" plane through (0, 0, 0) normal (0, 0, 1) x (1, 0, 0)
  arc A0 (-68.5, 131.4283) -> (-67.9, 131.6283) centre (-68.5, 132.4283) ccw projected
  arc A1 (-61.6309, 129.4431) -> (-67.9, 131.6283) centre (-65.5, 128.4283) ccw projected
  arc A2 (-61.6309, 129.4431) -> (-59.8309, 129.1431) centre (-60.6636, 129.6968) ccw projected
  arc A3 (-54.2, 123.6556) -> (-59.8309, 129.1431) centre (-56.5, 126.9283) ccw projected
  line L0 (-54.2, 123.6556) -> (-66.7, 114.8708) projected
  arc A4 (-71.5092, 115.0284) -> (-66.7, 114.8708) centre (-69, 118.1435) ccw projected
  line L1 (-71.5092, 115.0284) -> (-83.3819, 124.592) projected
  arc A5 (-79.1581, 128.8033) -> (-83.3819, 124.592) centre (-81.5, 126.9283) ccw projected
  arc A6 (-79.1581, 128.8033) -> (-78.3775, 128.4283) centre (-78.3775, 129.4283) ccw projected
  line L2 (-78.3775, 128.4283) -> (-77.399, 128.4283) projected
  arc A7 (-77.399, 128.4283) -> (-76.4192, 129.2283) centre (-77.399, 129.4283) ccw projected
  arc A8 (-70.1, 131.6283) -> (-76.4192, 129.2283) centre (-72.5, 128.4283) ccw projected
  arc A9 (-70.1, 131.6283) -> (-69.5, 131.4283) centre (-69.5, 132.4283) ccw projected
  line L3 (-69.5, 131.4283) -> (-68.5, 131.4283) projected
  arc A10 (-64.5, 128.4283) -> (-66.5, 128.4283) centre (-65.5, 128.4283) ccw projected
  line L4 (-66.5, 128.4283) -> (-71.5, 128.4283) projected
  arc A11 (-71.5, 128.4283) -> (-73.5, 128.4283) centre (-72.5, 128.4283) ccw projected
  line L5 (-73.5, 128.4283) -> (-73.5, 125.4283) projected
  arc A12 (-73.5, 125.4283) -> (-71.5, 125.4283) centre (-72.5, 125.4283) ccw projected
  line L6 (-71.5, 125.4283) -> (-66.5, 125.4283) projected
  arc A13 (-66.5, 125.4283) -> (-64.5, 125.4283) centre (-65.5, 125.4283) ccw projected
  line L7 (-64.5, 125.4283) -> (-64.5, 128.4283) projected
  circle A14 centre (-81.5, 126.9283) radius 1.5 projected
  circle A15 centre (-56.5, 126.9283) radius 1.5 projected
  circle A16 centre (-69, 118.1435) radius 1.5 projected
  line L8 (-67.5625, 116.0981) -> (-55.0625, 124.8829)
  arc A17 (-55.0625, 124.8829) -> (-58.5818, 128.3125) centre (-56.5, 126.9283) ccw
  arc A18 (-63.0818, 129.0625) -> (-58.5818, 128.3125) centre (-60.6636, 129.6968) ccw
  arc A19 (-63.0818, 129.0625) -> (-67, 130.4283) centre (-65.5, 128.4283) ccw
  arc A20 (-68.5, 129.9283) -> (-67, 130.4283) centre (-68.5, 132.4283) ccw
  line L9 (-68.5, 129.9283) -> (-69.5, 129.9283)
  arc A21 (-71, 130.4283) -> (-69.5, 129.9283) centre (-69.5, 132.4283) ccw
  arc A22 (-71, 130.4283) -> (-74.9495, 128.9283) centre (-72.5, 128.4283) ccw
  arc A23 (-77.399, 126.9283) -> (-74.9495, 128.9283) centre (-77.399, 129.4283) ccw
  line L10 (-77.399, 126.9283) -> (-78.3775, 126.9283)
  arc A24 (-80.3291, 127.8658) -> (-78.3775, 126.9283) centre (-78.3775, 129.4283) ccw
  arc A25 (-80.3291, 127.8658) -> (-82.441, 125.7601) centre (-81.5, 126.9283) ccw
  line L11 (-82.441, 125.7601) -> (-70.5683, 116.1965)
  arc A26 (-70.5683, 116.1965) -> (-67.5625, 116.0981) centre (-69, 118.1435) ccw
  circle A27 centre (-81.5, 126.9283) radius 3
  circle A28 centre (-69, 118.1435) radius 4
  circle A29 centre (-56.5, 126.9283) radius 4
  arc A30 (-61.5, 128.4283) -> (-68.1458, 131.4283) centre (-65.5, 128.4283) ccw
  line L12 (-68.1458, 131.4283) -> (-69.8542, 131.4283)
  arc A31 (-69.8542, 131.4283) -> (-76.5, 128.4283) centre (-72.5, 128.4283) ccw
  line L13 (-76.5, 128.4283) -> (-76.5, 125.4283)
  arc A32 (-76.5, 125.4283) -> (-69.8542, 122.4283) centre (-72.5, 125.4283) ccw
  line L14 (-69.8542, 122.4283) -> (-68.1458, 122.4283)
  arc A33 (-68.1458, 122.4283) -> (-61.5, 125.4283) centre (-65.5, 125.4283) ccw
  line L15 (-61.5, 125.4283) -> (-61.5, 128.4283)
  arc A34 (-72.5233, 120.0373) -> (-73.2233, 121.4942) centre (-73.4041, 120.5107) ccw
  arc A35 (-64.7767, 121.4942) -> (-65.4767, 120.0373) centre (-64.5959, 120.5107) ccw
  arc A36 (-59.8309, 124.7135) -> (-61.6309, 124.4135) centre (-60.6636, 124.1598) ccw
  point P0 (0, 0)
  point P1 (-78.5, 126.9313)
  point P2 (-80.4177, 124.1303)
  point P3 (-73, 118.1553)
  point P4 (-76.5, 127.0955)
  point P5 (-65.0078, 117.8935)
  point P6 (-57.6172, 123.0875)
  dimension "d40" = 1.5
  dimension "d41" = 3
  dimension "d42" = 2
  dimension "d43" = 2
  dimension "d44" = 2
  constraints: 42 point on circle, 19 centre point, 16 end point, 6 tangent, 3 coincident, 23 other
  measures "d40" distance between parallel lines of L0 L8
  measures "d41" distance between parallel lines of L7 L15
  measures "d42" diameter of A34
  measures "d43" diameter of A35
  measures "d44" diameter of A36
extrude "押し出し8" cut sketch "スケッチ5" against normal blind 2.5 contours A29 L8 A28 A35 A33 A36 | L13 A32 A34 A28 L11 A27 A24 L10 A23
fillet "フィレット3" radius 1 6 edges at (-78.5, 126.9313, -1.25) (-76.5, 127.0955, -1.25) (-80.4177, 124.1303, -1.25) (-73, 118.1553, -1.25) (-65.0078, 117.8935, -1.25) (-57.6172, 123.0875, -1.25)
